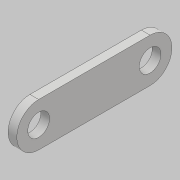
# Autodesk Inventor part: exercise3-20ipt
Saved by Autodesk Inventor 2018 (Build 220112000, 112)
## iProperties
Created: 2020-09-23
Part Number: exercise3-20ipt
Material: 一般
Document SubType Name: Modeling
Designer: 王鼎鈞
Density: 1 g/cm^3
Appearance: 預設
Author: 王鼎鈞
Autodesk Inventor part; units mm, degrees
ref_plane "YZ Plane" through (0, 0, 0) normal (1, 0, 0) x (0, 1, 0)
ref_plane "XZ Plane" through (0, 0, 0) normal (0, 1, 0) x (-1, 0, 0)
ref_plane "XY Plane" through (0, 0, 0) normal (0, 0, 1) x (1, 0, 0)
sketch "草圖1" plane through (0, 0, 0) normal (1, 0, 0) x (0, 1, 0)
  line L0 (-127.5, 0) -> (127.5, 0) construction
  line L1 (-127.5, -50) -> (127.5, -50)
  line L2 (127.5, 50) -> (-127.5, 50)
  arc A0 (-127.5, 50) -> (-127.5, -50) centre (-127.5, 0) ccw
  arc A1 (127.5, -50) -> (127.5, 50) centre (127.5, 0) ccw
  circle A2 centre (127.5, 0) radius 25
  circle A3 centre (-127.5, 0) radius 25
  point P0 (0, 0)
  dimension "d0" = 127.5
  dimension "d1" = 100
  dimension "d2" = 50
  dimension "d3" = 50
  constraints: 8 end point, 4 centre point, 4 point on circle, 4 tangent, 2 coincident, 1 horizontal, 1 midpoint, 1 parallel
  measures "d0" distance of point (0, 0) L0.end
  measures "d1" diameter of A1
  measures "d2" diameter of A2
  measures "d3" diameter of A3
extrude "擠出1" add sketch "草圖1" along normal blind 20
